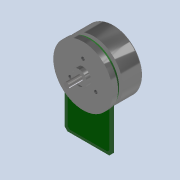
# Autodesk Inventor part: MaxonEC45-50W-MILE
Saved by Autodesk Inventor 2020.4 (Build 244396000, 396)
## iProperties
Created: 2015-08-10
Part Number: MaxonEC45-50W-MILE
Material: Edelstahl
Document SubType Name: Modeling
Designer: ryll
Mass: 275.995 g
Surface Area: 92.5658 cm^2
Volume: 34.4994 cm^3
Density: 8 g/cm^3
Appearance: Halbpoliert
Author: ryll
Autodesk Inventor part; units mm, degrees
ref_plane "YZ Plane" through (0, 0, 0) normal (1, 0, 0) x (0, 1, 0)
ref_plane "XZ Plane" through (0, 0, 0) normal (0, 1, 0) x (-1, 0, 0)
ref_plane "XY Plane" through (0, 0, 0) normal (0, 0, 1) x (1, 0, 0)
sketch "Skizze1" plane through (0, 0, 0) normal (1, 0, 0) x (0, 1, 0)
  line L0 (0, 26.4) -> (0, -4.4) projected
  line L1 (0, 6) -> (0, 22)
  line L2 (0, 22) -> (4, 22)
  line L3 (4, 22) -> (4, 21.2)
  line L4 (4, 21.2) -> (5.6, 21.2)
  line L5 (5.6, 21.2) -> (5.6, 18.25)
  line L6 (5.6, 18.25) -> (7.7, 18.25)
  line L7 (7.7, 18.25) -> (7.7, 21.7)
  line L8 (7.7, 21.7) -> (22.6, 21.7)
  line L9 (22.6, 21.7) -> (22.6, 0)
  line L10 (-20.2, 0) -> (22.6, 0) construction
  line L11 (0, 6) -> (-3.2, 6)
  line L12 (-3.2, 6) -> (-3.2, 2)
  line L13 (-3.2, 2) -> (-20.2, 2)
  line L14 (-20.2, 2) -> (-20.2, 0)
  line L15 (-28.76, 0) -> (31.16, 0) projected
  line L16 (-20.2, 0) -> (22.6, 0)
  point P0 (0, 0)
  dimension "d0" = 44
  dimension "d1" = 4
  dimension "d2" = 1.6
  dimension "d3" = 2.1
  dimension "d4" = 22.6
  dimension "d5" = 43.4
  dimension "d6" = 12
  dimension "d7" = 4
  dimension "d8" = 3.2
  dimension "d9" = 20.2
  dimension "d10" = 42.4
  dimension "d11" = 36.5
  constraints: 30 end point, 9 perpendicular, 3 collinear, 3 horizontal, 1 vertical
  measures "d0" diameter of L2 L10
  measures "d1" distance of L1.end L2.end
  measures "d2" distance of L3.end L4.end
  measures "d3" distance of L5.end L6.end
  measures "d4" distance between parallel lines of L1 L9
  measures "d5" diameter of L8 L10
  measures "d6" diameter of L11 L10
  measures "d7" diameter of L13 L10
  measures "d8" distance of L1.start L11.end
  measures "d9" distance between parallel lines of L1 L14
  measures "d10" diameter of L4 L10
  measures "d11" diameter of L6 L10
revolve "Umdrehung1" add sketch "Skizze1" angle 360 about axis through (0, -20.2, 0) along (0, 1, 0)
fillet "Rundung1" radius 1 1 edges at (0, 22.6, -21.7)
sketch "Skizze2" plane through (0, -3.2, 0) normal (0, -1, 0) x (1, 0, 0)
  circle A0 centre (0, 0) radius 6 projected
  circle A1 centre (0, 0) radius 5
  circle A2 centre (0, 0) radius 2
  dimension "d14" = 1
  constraints: 2 centre point, 2 coincident
  measures "d14" radial gap between concentric circles of A0 A1
extrude "Extrusion1" cut sketch "Skizze2" against normal blind 1 contours A1
sketch "Skizze3" plane through (0, 0, 0) normal (0, -1, 0) x (1, 0, 0)
  line L0 (0, 30.8) -> (0, -30.8) projected
  line L1 (-30.8, 0) -> (30.8, 0) projected
  point P0 (0, 0)
  point P1 (0, 11)
  dimension "d17" = 11
  constraints: 1 point on line
  measures "d17" distance from line of point (0, 11) L1
hole "Bohrung1" at (0, 0, 11) direction (0, 1, 0) diameter 2.459 depth 3.9 tip angle 118 thread size "M3x0.5" class "6H" standard "ANSI Metric M Profile"
pattern_circular "Runde Anordnung1" count 3 over 360 about axis through (0, -10, 0) along (0, 1, 0) of "Bohrung1"
sketch "Skizze4" plane through (0, 5.6, 0) normal (0, 1, 0) x (1, 0, 0)
  line L0 (30.8, 0) -> (-30.8, 0) projected
  circle A0 centre (0, 0) radius 21.2 projected
  line L1 (-17.5, 11.9662) -> (-17.5, 45.3)
  line L2 (-17.5, 45.3) -> (17.5, 45.3)
  line L3 (17.5, 45.3) -> (17.5, 11.9662)
  arc A1 (17.5, 11.9662) -> (-17.5, 11.9662) centre (0, 0) ccw
  line L4 (0, 52.3131) -> (0, -34.3855) projected
  dimension "d28" = 35
  dimension "d29" = 45.3
  constraints: 6 end point, 4 point on circle, 2 parallel, 1 centre point, 1 concentric, 1 other
  measures "d28" distance of L1.end L2.end
  measures "d29" distance between parallel lines of L2 L0
extrude "Extrusion2" add sketch "Skizze4" against normal blind 1.6 contours A0 L4 L2 L3 | A0 L1 L2 L4
chamfer "Fase1" distance 2 angle 45 2 edges at (17.5, 4.8, -45.3) (-17.5, 4.8, -45.3)
sketch "Sketch5" plane through (0, 4, 0) normal (0, -1, 0) x (1, 0, 0)
  line L0 (-17.5, -43.3) -> (-15.5, -45.3) projected
  line L1 (-17.5, -43.3) -> (-17.5, -11.9662) projected
  arc A0 (17.5, -11.9662) -> (-17.5, -11.9662) centre (0, 0) ccw projected
  line L2 (17.5, -11.9662) -> (17.5, -43.3) projected
  line L3 (15.5, -45.3) -> (17.5, -43.3) projected
  line L4 (15.5, -45.3) -> (-15.5, -45.3) projected
  circle A1 centre (0, 0) radius 18.25 projected
  line L5 (17.5, -11.9662) -> (15.5, -11.9662)
  line L6 (15.5, -11.9662) -> (15.5, -41.9662)
  line L7 (15.5, -41.9662) -> (14.0858, -43.3804)
  line L8 (14.0858, -43.3804) -> (-13.9142, -43.3804)
  line L9 (-13.9142, -43.3804) -> (-15.3284, -41.9662)
  line L10 (-15.3284, -41.9662) -> (-15.3284, -11.9662)
  line L11 (-15.3284, -11.9662) -> (-17.5, -11.9662)
  dimension "d35" = 2
  dimension "d36" = 30
  dimension "d37" = 2
  dimension "d38" = 135
  dimension "d39" = 28
  dimension "d40" = 135
  dimension "d41" = 2
  dimension "d42" = 135
  constraints: 14 end point, 3 perpendicular, 2 parallel, 1 horizontal, 1 point on line
  measures "d35" distance of L2.start L5.end
  measures "d36" distance of L5.end L6.end
  measures "d37" distance of L6.end L7.end
  measures "d38" angle of L6 L7
  measures "d39" distance of L7.end L8.end
  measures "d40" angle of L7 L8
  measures "d41" distance of L8.end L9.end
  measures "d42" angle of L8 L9
extrude "Extrusion3" cut sketch "Sketch5" against normal blind 0.01 contours L1 L11 L10 L9 L8 L7 L6 L5 L2 L3 L4 L0
sketch "Sketch6" plane through (0, -20.2, 0) normal (0, -1, 0) x (1, 0, 0)
  circle A0 centre (0, 0) radius 2 projected
extrude "Extrusion4" cut sketch "Sketch6" against normal blind 8
